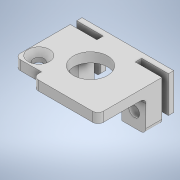
# Autodesk Inventor part: switch-mount
Saved by Autodesk Inventor 2021 (Build 250183000, 183)
## iProperties
Created: 2024-05-22
Part Number: switch-mount
Material: Generic
Document SubType Name: Modeling
Designer: Toby
Density: 1 g/cm^3
Appearance: Default
Author: Toby
Autodesk Inventor part; units mm, degrees
ref_plane "YZ Plane" through (0, 0, 0) normal (1, 0, 0) x (0, 1, 0)
ref_plane "XZ Plane" through (0, 0, 0) normal (0, 1, 0) x (-1, 0, 0)
ref_plane "XY Plane" through (0, 0, 0) normal (0, 0, 1) x (1, 0, 0)
sketch "Sketch1" plane through (0, 0, 0) normal (0, 0, 1) x (1, 0, 0)
  line L0 (-2.358, 4.2713) -> (4.842, 4.2713)
  line L1 (4.842, 4.2713) -> (4.842, 2.2713)
  line L2 (4.842, 2.2713) -> (-2.358, 2.2713)
  line L3 (-2.358, 2.2713) -> (-2.358, 4.2713)
  line L4 (-2.358, 4.2713) -> (-7.358, 4.2713)
  line L5 (-7.358, 4.2713) -> (-7.358, -3.7287)
  line L6 (-7.358, -3.7287) -> (-2.358, -3.7287)
  line L7 (-2.358, -3.7287) -> (-2.358, 4.2713)
  line L8 (4.842, 4.2713) -> (9.842, 4.2713)
  line L9 (9.842, 4.2713) -> (9.842, -3.7287)
  line L10 (9.842, -3.7287) -> (4.842, -3.7287)
  line L11 (4.842, -3.7287) -> (4.842, 4.2713)
  point P0 (0, 0)
  point P1 (-2.358, 2.2713)
  point P2 (4.842, 2.2713)
  point P3 (-2.358, 2.2713)
  dimension "d0" = 7.2
  dimension "d1" = 2
  dimension "d2" = 8
  dimension "d3" = 5
  dimension "d4" = 5
  constraints: 24 end point, 6 parallel, 3 horizontal, 3 perpendicular, 1 point on line
  measures "d0" distance of L1.end L2.end
  measures "d1" distance between parallel lines of L2 L0
  measures "d2" distance between parallel lines of L6 L4
  measures "d3" distance between parallel lines of L7 L5
  measures "d4" distance of L0.end L8.end
extrude "Extrusion1" add sketch "Sketch1" along normal blind 12
sketch "Sketch2" plane through (0, 0, 0) normal (0, 0, -1) x (-1, 0, 0)
  line L0 (2.358, 2.2713) -> (-4.842, 2.2713) projected
  line L1 (-9.842, 4.2713) -> (7.358, 4.2713) projected
  line L2 (2.358, 2.2713) -> (-4.842, 2.2713)
  line L3 (-4.842, 2.2713) -> (-4.842, 4.2713)
  line L4 (-4.842, 4.2713) -> (2.358, 4.2713)
  line L5 (2.358, 4.2713) -> (2.358, 2.2713)
  line L6 (-4.842, 2.2713) -> (-4.842, -3.7287) projected
  point P0 (0, 0)
  point P1 (-4.842, 2.2713)
  constraints: 8 end point, 2 parallel, 1 collinear, 1 horizontal, 1 perpendicular, 1 point on line
extrude "Extrusion2" add sketch "Sketch2" along normal blind 1.2
sketch "Sketch3" plane through (0, 0, -1.2) normal (0, 0, -1) x (-1, 0, 0)
  line L0 (-9.842, -3.7287) -> (-9.842, 4.2713) projected
  line L1 (7.358, 4.2713) -> (7.358, -3.7287) projected
  line L2 (-9.842, 4.2713) -> (7.358, 4.2713)
  line L3 (7.358, 4.2713) -> (7.358, -3.7287)
  line L4 (7.358, -3.7287) -> (-9.842, -3.7287)
  line L5 (-9.842, -3.7287) -> (-9.842, 4.2713)
  point P0 (0, 0)
  constraints: 8 end point, 2 parallel, 1 horizontal, 1 perpendicular
extrude "Extrusion3" add sketch "Sketch3" along normal blind 1
sketch "Sketch4" plane through (0, 0, 12) normal (0, 0, 1) x (1, 0, 0)
  line L0 (-7.358, -3.7287) -> (-7.358, 4.2713) projected
  line L1 (9.842, 4.2713) -> (9.842, -3.7287) projected
  line L2 (-7.358, 2.2713) -> (9.842, 2.2713)
  line L3 (9.842, 2.2713) -> (9.842, -3.7287)
  line L4 (9.842, -3.7287) -> (-7.358, -3.7287)
  line L5 (-7.358, -3.7287) -> (-7.358, 2.2713)
  line L6 (-2.358, 2.2713) -> (4.842, 2.2713) projected
  point P0 (0, 0)
  constraints: 8 end point, 2 parallel, 1 collinear, 1 horizontal, 1 perpendicular, 1 point on line
extrude "Extrusion4" cut sketch "Sketch4" against normal blind 9
sketch "Sketch5" plane through (0, 0, 3) normal (0, 0, 1) x (1, 0, 0)
  line L0 (9.842, 4.2713) -> (-7.358, 4.2713) projected
  line L1 (-2.358, 2.2713) -> (-2.358, -3.7287) projected
  line L2 (4.842, -3.7287) -> (4.842, 2.2713) projected
  point P0 (0, 0)
  point P1 (-5.358, -1.0287)
  point P2 (7.642, -1.0287)
  dimension "d13" = 5.3
  dimension "d14" = 3
  dimension "d15" = 5.3
  dimension "d16" = 2.8
  measures "d13" distance from line of L0 point (-5.358, -1.029)
  measures "d14" distance from line of L1 point (-5.358, -1.029)
  measures "d15" distance from line of L0 point (7.642, -1.029)
  measures "d16" distance from line of L2 point (7.642, -1.029)
hole "Hole1" at (-5.358, -1.0287, 3) at (7.642, -1.0287, 3) direction (0, 0, -1) diameter 2 depth 5 tip angle 118
sketch "Sketch6" plane through (0, 0, -1.2) normal (0, 0, 1) x (1, 0, 0)
  line L0 (-2.358, 2.2713) -> (-2.358, -3.7287) projected
  line L1 (4.842, 2.2713) -> (4.842, -3.7287) projected
  line L2 (-2.358, 2.2713) -> (4.842, 2.2713)
  line L3 (4.842, 2.2713) -> (4.842, -3.7287)
  line L4 (4.842, -3.7287) -> (-2.358, -3.7287)
  line L5 (-2.358, -3.7287) -> (-2.358, 2.2713)
  point P0 (0, 0)
  point P1 (4.842, 2.2713)
  constraints: 8 end point, 2 parallel, 1 horizontal, 1 perpendicular
extrude "Extrusion5" cut sketch "Sketch6" against normal blind 2
sketch "Sketch7" plane through (-7.358, 4.2713, 12) normal (0, 1, 0) x (1, 0, 0)
  line L0 (0, 14.2) -> (17.2, 14.2) projected
  line L1 (17.2, 12) -> (17.2, 0) projected
  line L2 (0, 14.2) -> (17.2, 14.2)
  line L3 (17.2, 14.2) -> (17.2, 0)
  line L4 (17.2, 0) -> (0, 0)
  line L5 (0, 0) -> (0, 14.2)
  point P0 (7.358, 12)
  constraints: 8 end point, 2 parallel, 1 horizontal, 1 perpendicular
extrude "Extrusion6" cut sketch "Sketch7" against normal blind 0.2
sketch "Sketch8" plane through (-7.358, 4.0713, 12) normal (0, 1, 0) x (1, 0, 0)
  line L0 (0, 14.2) -> (17.2, 14.2) projected
  circle A0 centre (8.6, 7.2) radius 3.2
  point P0 (7.358, 12)
  dimension "d31" = 7
  dimension "d32" = 6.4
  constraints: 1 centre point, 1 coincident
  measures "d31" distance from line of point (8.6, 7.2) L0
  measures "d32" diameter of A0
extrude "Extrusion7" cut sketch "Sketch8" against normal blind 2
sketch "Sketch9" plane through (-7.358, 4.0713, 12) normal (0, 1, 0) x (1, 0, 0)
  line L0 (0, 9) -> (0, 0) projected
  line L1 (0, 0) -> (17.2, 0) projected
  line L2 (0, 1.6) -> (5, 1.6)
  line L3 (5, 1.6) -> (5, 0)
  line L4 (5, 0) -> (0, 0)
  line L5 (0, 0) -> (0, 1.6)
  point P0 (7.358, 12)
  dimension "d35" = 1.6
  dimension "d36" = 5
  constraints: 8 end point, 2 parallel, 2 point on line, 1 horizontal, 1 perpendicular
  measures "d35" distance between parallel lines of L1 L2
  measures "d36" distance between parallel lines of L0 L3
extrude "Extrusion8" cut sketch "Sketch9" against normal blind 2
fillet "Fillet1" radius 1 2 edges at (-4.858, 2.2713, 3) (7.342, 2.2713, 3)
fillet "Fillet2" radius 1 3 edges at (-7.358, 3.1713, 10.4) (9.842, 3.1713, 12) (-2.358, 3.1713, 12)
sketch "Sketch10" plane through (0, 0, -2.2) normal (0, 0, -1) x (-1, 0, 0)
  line L0 (7.358, -3.7287) -> (2.358, -3.7287) projected
  line L1 (-9.842, 4.0713) -> (-9.842, -3.7287) projected
  line L2 (7.358, -3.7287) -> (-9.842, -3.7287)
  line L3 (-9.842, -3.7287) -> (-9.842, -2.7287)
  line L4 (-9.842, -2.7287) -> (7.358, -2.7287)
  line L5 (7.358, -2.7287) -> (7.358, -3.7287)
  point P0 (0, 0)
  point P1 (-9.842, -3.7287)
  point P2 (2.358, -3.7287)
  dimension "d45" = 1
  constraints: 8 end point, 2 parallel, 1 horizontal, 1 perpendicular, 1 point on line
  measures "d45" distance between parallel lines of L4 L0
extrude "Extrusion9" cut sketch "Sketch10" against normal blind 1
fillet "Fillet4" radius 1 2 edges at (-7.358, -3.7287, 1.5) (9.842, -3.7287, 1.5)
chamfer "Chamfer3" distance 1 angle 45 2 edges at (-2.358, -2.7287, -1.7) (4.842, -2.7287, -1.7)
sketch "Sketch11" plane through (0, 0, -2.2) normal (0, 0, -1) x (-1, 0, 0)
  line L0 (-9.842, 2.2713) -> (-4.842, 2.2713) projected
  line L1 (-5.342, 2.2713) -> (2.858, 2.2713)
  line L2 (2.858, 2.2713) -> (2.858, -3.7287)
  line L3 (2.858, -3.7287) -> (-5.342, -3.7287)
  line L4 (-5.342, -3.7287) -> (-5.342, 2.2713)
  line L5 (-4.842, -1.7287) -> (-4.842, 2.2713) projected
  line L6 (2.358, 2.2713) -> (2.358, -1.7287) projected
  line L7 (-4.842, -3.7287) -> (-8.842, -3.7287) projected
  point P0 (0, 0)
  dimension "d52" = 8.2
  dimension "d53" = 0.5
  dimension "d54" = 0.5
  constraints: 8 end point, 2 parallel, 1 collinear, 1 horizontal, 1 perpendicular, 1 point on line
  measures "d52" distance of L2.end L3.end
  measures "d53" distance between parallel lines of L5 L4
  measures "d54" distance between parallel lines of L6 L2
extrude "Extrusion10" cut sketch "Sketch11" against normal blind 10
sketch "Sketch12" plane through (-7.358, 4.0713, 12) normal (0, 1, 0) x (1, 0, 0)
  line L0 (0, 2.6) -> (0, 12) projected
  line L1 (1, 1.6) -> (5, 1.6) projected
  point P0 (7.358, 12)
  point P1 (2.1, 4)
  dimension "d57" = 2.1
  dimension "d58" = 2.4
  measures "d57" distance from line of L0 point (2.1, 4)
  measures "d58" distance from line of L1 point (2.1, 4)
hole "Hole2" at (-5.258, 4.0713, 8) direction (0, -1, 0) diameter 2 depth 5 tip angle 118 countersink diameter 4 countersink angle 90
body "Solid1"
